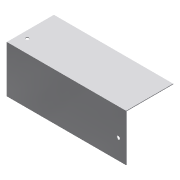
# Autodesk Inventor part: L profil
Saved by Autodesk Inventor 2015 (Build 190159000, 159)
## iProperties
Created: 2015-01-07
Part Number: L profil
Material: Všeobecné
Document SubType Name: Modeling
Designer: Michal
Density: 1 g/cm^3
Appearance: Hliník – leštěný
Author: Michal
Autodesk Inventor part; units mm, degrees
ref_plane "YZ Plane" through (0, 0, 0) normal (1, 0, 0) x (0, 1, 0)
ref_plane "XZ Plane" through (0, 0, 0) normal (0, 1, 0) x (-1, 0, 0)
ref_plane "XY Plane" through (0, 0, 0) normal (0, 0, 1) x (1, 0, 0)
sketch "Náčrt1" plane through (0, 0, 0) normal (1, 0, 0) x (0, 1, 0)
  line L0 (0, 0) -> (150, 0)
  line L1 (150, 0) -> (150, -2)
  line L2 (150, -2) -> (2, -2)
  line L3 (2, -2) -> (2, -150)
  line L4 (2, -150) -> (0, -150)
  line L5 (0, -150) -> (0, 0)
  point P0 (150, -148)
  point P1 (150, -150)
  dimension "d0" = 150
  dimension "d1" = 2
  dimension "d20" = 150
  dimension "d21" = 148
  constraints: 12 end point, 3 perpendicular, 2 point on line, 1 horizontal
  measures "d0" distance of L0.start L0.end
  measures "d1" distance of L0.end L1.end
  measures "d20" distance of L4.end L0.start
  measures "d21" distance of L1.end L2.end
extrude "Vysunutí1" add sketch "Náčrt1" along normal blind 380
sketch "Náčrt4" plane through (0, 2, -2) normal (0, 1, 0) x (1, 0, 0)
  line L0 (0, 0) -> (0, 148) projected
  line L1 (0, 0) -> (380, 0) projected
  line L2 (380, 148) -> (380, 0) projected
  circle A0 centre (355, 85) radius 5.25
  line L3 (0, 148) -> (380, 148) projected
  line L4 (0, 148) -> (0, -2) projected
  line L5 (0, 148) -> (380, 148) projected
  line L6 (380, -2) -> (380, 148) projected
  line L7 (0, -2) -> (380, -2) projected
  dimension "d14" = 25
  dimension "d16" = 10.5
  dimension "d39" = 87
  constraints: 1 centre point
  measures "d14" distance from line of L2 A0.centre
  measures "d16" diameter of A0
  measures "d39" distance from line of A0.centre L7
extrude "Vysunutí3" cut sketch "Náčrt4" against normal through all contours A0
sketch "Náčrt5" plane through (0, 0, 0) normal (0, 0, 1) x (1, 0, 0)
  circle A0 centre (23, 42) radius 5.25
  line L0 (380, 150) -> (380, 0) projected
  line L1 (0, 0) -> (380, 0) projected
  dimension "d22" = 10.5
  dimension "d23" = 357
  dimension "d24" = 42
  constraints: 1 centre point
  measures "d22" diameter of A0
  measures "d23" distance from line of L0 A0.centre
  measures "d24" distance from line of L1 A0.centre
extrude "Vysunutí4" cut sketch "Náčrt5" against normal through all
